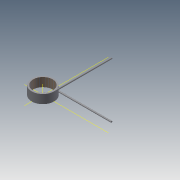
# Autodesk Inventor part: TOS 0.3-4-270-5
Saved by Autodesk Inventor 2015 SP1 (Build 190203100, 203)
## iProperties
Created: 2015-02-17
Part Number: TOS 0.3-4-270-5
Material: 一般
Document SubType Name: Modeling
Designer: Yamaura
Density: 1 g/cm^3
Appearance: 既定
Author: Yamaura
Autodesk Inventor part; units mm, degrees
ref_plane "YZ Plane" through (0, 0, 0) normal (1, 0, 0) x (0, 1, 0)
ref_plane "XZ Plane" through (0, 0, 0) normal (0, 1, 0) x (-1, 0, 0)
ref_plane "XY Plane" through (0, 0, 0) normal (0, 0, 1) x (1, 0, 0)
sketch "スケッチ1" plane through (0, 0, 0) normal (0, 0, 1) x (1, 0, 0)
  circle A0 centre (0, 0) radius 2
  dimension "d0" = 4
  constraints: 1 centre point, 1 coincident
  measures "d0" diameter of A0
surface extrude "押し出しサーフェス1" sketch "スケッチ1" along normal blind 1.8 shown yes curves A0
thicken "厚み1" operation new thickness 0.3 both sides no extend neighbours no toward (0.9870503, -0.1604113, 0) faces at (1.9741, -0.3208, 1.2)
sketch "スケッチ2" plane through (0, 0, 0) normal (1, 0, 0) x (0, 1, 0)
  circle A0 centre (2.15, 0.15) radius 0.15
  line L0 (2.3, 0) -> (-2.3, 0) projected
  line L1 (0, -0.1) -> (0, 0.6) projected
  point P0 (0, 0)
  dimension "d5" = 0.3
  dimension "d6" = 0.15
  dimension "d7" = 2.15
  constraints: 1 centre point
  measures "d5" diameter of A0
  measures "d6" distance from line of A0.centre L0
  measures "d7" distance from line of L1 A0.centre
extrude "押し出し1" add sketch "スケッチ2" along normal blind 12
sketch "スケッチ3" plane through (0, 0, 0) normal (0, 1, 0) x (-1, 0, 0)
  circle A0 centre (-2.15, 1.65) radius 0.15
  line L0 (2.3, 0) -> (-2.3, 0) projected
  line L1 (0, -0.464) -> (0, 2.7607) projected
  point P0 (0, 0)
  point P1 (-0.817, 0)
  dimension "d10" = 0.3
  dimension "d11" = 1.65
  dimension "d12" = 2.15
  constraints: 1 centre point
  measures "d10" diameter of A0
  measures "d11" distance from line of A0.centre L0
  measures "d12" distance from line of L1 A0.centre
extrude "押し出し2" add sketch "スケッチ3" along normal blind 12
